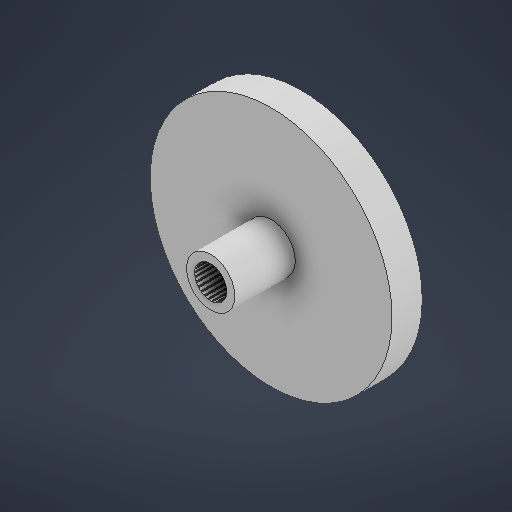
# Autodesk Inventor part: Part7
Saved by Autodesk Inventor 2026.2 (Build 302298000, 298)
## iProperties
Created: 2026-04-16
Part Number: Part7
Material: Generic
Document SubType Name: Modeling
Designer: danda
Density: 1 g/cm^3
Appearance: Default
Author: danda
Autodesk Inventor part; units mm, degrees
ref_plane "YZ Plane" through (0, 0, 0) normal (1, 0, 0) x (0, 1, 0)
ref_plane "XZ Plane" through (0, 0, 0) normal (0, 1, 0) x (-1, 0, 0)
ref_plane "XY Plane" through (0, 0, 0) normal (0, 0, 1) x (1, 0, 0)
sketch "Sketch1" plane through (0, 0, 0) normal (0, 0, 1) x (1, 0, 0)
  line L0 (27.0225, 22.9586) -> (27.3991, 23.1435)
  line L1 (27.3991, 23.1435) -> (27.4189, 23.2234)
  arc A0 (27.4189, 23.2234) -> (27.5041, 23.2788) centre (26.0453, 25.431) ccw
  line L2 (27.5041, 23.2788) -> (27.5858, 23.2643)
  line L3 (27.5858, 23.2643) -> (27.9072, 23.534)
  line L4 (27.9072, 23.534) -> (27.9073, 23.6163)
  arc A1 (27.9073, 23.6163) -> (27.9768, 23.6905) centre (26.0453, 25.431) ccw
  line L5 (27.9768, 23.6905) -> (28.0596, 23.6959)
  line L6 (28.0596, 23.6959) -> (28.3071, 24.0347)
  line L7 (28.3071, 24.0347) -> (28.2875, 24.1147)
  arc A2 (28.2875, 24.1147) -> (28.3372, 24.2033) centre (26.0453, 25.431) ccw
  line L8 (28.3372, 24.2033) -> (28.4163, 24.2284)
  line L9 (28.4163, 24.2284) -> (28.5755, 24.6165)
  line L10 (28.5755, 24.6165) -> (28.5373, 24.6895)
  arc A3 (28.5373, 24.6895) -> (28.5644, 24.7874) centre (26.0453, 25.431) ccw
  line L11 (28.5644, 24.7874) -> (28.6352, 24.8308)
  line L12 (28.6352, 24.8308) -> (28.6969, 25.2457)
  line L13 (28.6969, 25.2457) -> (28.6423, 25.3074)
  arc A4 (28.6423, 25.3074) -> (28.6452, 25.409) centre (26.0453, 25.431) ccw
  line L14 (28.6452, 25.409) -> (28.7035, 25.468)
  line L15 (28.7035, 25.468) -> (28.6642, 25.8857)
  line L16 (28.6642, 25.8857) -> (28.5964, 25.9326)
  arc A5 (28.5964, 25.9326) -> (28.5749, 26.0318) centre (26.0453, 25.431) ccw
  line L17 (28.5749, 26.0318) -> (28.6174, 26.1031)
  line L18 (28.6174, 26.1031) -> (28.4792, 26.4992)
  line L19 (28.4792, 26.4992) -> (28.4023, 26.5285)
  arc A6 (28.4023, 26.5285) -> (28.3576, 26.6197) centre (26.0453, 25.431) ccw
  line L20 (28.3576, 26.6197) -> (28.3818, 26.6991)
  line L21 (28.3818, 26.6991) -> (28.1529, 27.0507)
  line L22 (28.1529, 27.0507) -> (28.0711, 27.0607)
  arc A7 (28.0711, 27.0607) -> (28.0059, 27.1386) centre (26.0453, 25.431) ccw
  line L23 (28.0059, 27.1386) -> (28.0105, 27.2214)
  line L24 (28.0105, 27.2214) -> (27.704, 27.508)
  line L25 (27.704, 27.508) -> (27.6222, 27.4981)
  arc A8 (27.6222, 27.4981) -> (27.5403, 27.5582) centre (26.0453, 25.431) ccw
  line L26 (27.5403, 27.5582) -> (27.5249, 27.6397)
  line L27 (27.5249, 27.6397) -> (27.1587, 27.8446)
  line L28 (27.1587, 27.8446) -> (27.0817, 27.8155)
  arc A9 (27.0817, 27.8155) -> (26.9878, 27.8541) centre (26.0453, 25.431) ccw
  line L29 (26.9878, 27.8541) -> (26.9533, 27.9296)
  line L30 (26.9533, 27.9296) -> (26.5488, 28.0409)
  line L31 (26.5488, 28.0409) -> (26.4809, 27.9942)
  arc A10 (26.4809, 27.9942) -> (26.3805, 28.0093) centre (26.0453, 25.431) ccw
  line L32 (26.3805, 28.0093) -> (26.3289, 28.0743)
  line L33 (26.3289, 28.0743) -> (25.9095, 28.0856)
  line L34 (25.9095, 28.0856) -> (25.8548, 28.024)
  arc A11 (25.8548, 28.024) -> (25.7537, 28.0145) centre (26.0453, 25.431) ccw
  line L35 (25.7537, 28.0145) -> (25.6881, 28.0654)
  line L36 (25.6881, 28.0654) -> (25.2782, 27.9759)
  line L37 (25.2782, 27.9759) -> (25.2398, 27.903)
  arc A12 (25.2398, 27.903) -> (25.1439, 27.8697) centre (26.0453, 25.431) ccw
  line L38 (25.1439, 27.8697) -> (25.068, 27.9033)
  line L39 (25.068, 27.9033) -> (24.6914, 27.7184)
  line L40 (24.6914, 27.7184) -> (24.6716, 27.6385)
  arc A13 (24.6716, 27.6385) -> (24.5864, 27.5831) centre (26.0453, 25.431) ccw
  line L41 (24.5864, 27.5831) -> (24.5047, 27.5976)
  line L42 (24.5047, 27.5976) -> (24.1833, 27.3279)
  line L43 (24.1833, 27.3279) -> (24.1833, 27.2456)
  arc A14 (24.1833, 27.2456) -> (24.1138, 27.1714) centre (26.0453, 25.431) ccw
  line L44 (24.1138, 27.1714) -> (24.031, 27.166)
  line L45 (24.031, 27.166) -> (23.7835, 26.8272)
  line L46 (23.7835, 26.8272) -> (23.8031, 26.7472)
  arc A15 (23.8031, 26.7472) -> (23.7534, 26.6586) centre (26.0453, 25.431) ccw
  line L47 (23.7534, 26.6586) -> (23.6743, 26.6335)
  line L48 (23.6743, 26.6335) -> (23.5151, 26.2454)
  line L49 (23.5151, 26.2454) -> (23.5532, 26.1724)
  arc A16 (23.5532, 26.1724) -> (23.5262, 26.0745) centre (26.0453, 25.431) ccw
  line L50 (23.5262, 26.0745) -> (23.4554, 26.0311)
  line L51 (23.4554, 26.0311) -> (23.3937, 25.6162)
  line L52 (23.3937, 25.6162) -> (23.4482, 25.5545)
  arc A17 (23.4482, 25.5545) -> (23.4454, 25.4529) centre (26.0453, 25.431) ccw
  line L53 (23.4454, 25.4529) -> (23.387, 25.3939)
  line L54 (23.387, 25.3939) -> (23.4264, 24.9762)
  line L55 (23.4264, 24.9762) -> (23.4941, 24.9293)
  arc A18 (23.4941, 24.9293) -> (23.5157, 24.8301) centre (26.0453, 25.431) ccw
  line L56 (23.5157, 24.8301) -> (23.4731, 24.7588)
  line L57 (23.4731, 24.7588) -> (23.6113, 24.3627)
  line L58 (23.6113, 24.3627) -> (23.6883, 24.3334)
  arc A19 (23.6883, 24.3334) -> (23.733, 24.2422) centre (26.0453, 25.431) ccw
  line L59 (23.733, 24.2422) -> (23.7087, 24.1628)
  line L60 (23.7087, 24.1628) -> (23.9377, 23.8112)
  line L61 (23.9377, 23.8112) -> (24.0195, 23.8012)
  arc A20 (24.0195, 23.8012) -> (24.0847, 23.7233) centre (26.0453, 25.431) ccw
  line L62 (24.0847, 23.7233) -> (24.0801, 23.6405)
  line L63 (24.0801, 23.6405) -> (24.3866, 23.3539)
  line L64 (24.3866, 23.3539) -> (24.4683, 23.3638)
  arc A21 (24.4683, 23.3638) -> (24.5503, 23.3037) centre (26.0453, 25.431) ccw
  line L65 (24.5503, 23.3037) -> (24.5657, 23.2222)
  line L66 (24.5657, 23.2222) -> (24.9318, 23.0173)
  line L67 (24.9318, 23.0173) -> (25.0089, 23.0464)
  arc A22 (25.0089, 23.0464) -> (25.1028, 23.0078) centre (26.0453, 25.431) ccw
  line L68 (25.1028, 23.0078) -> (25.1373, 22.9323)
  line L69 (25.1373, 22.9323) -> (25.5418, 22.821)
  line L70 (25.5418, 22.821) -> (25.6096, 22.8677)
  arc A23 (25.6096, 22.8677) -> (25.7101, 22.8526) centre (26.0453, 25.431) ccw
  line L71 (25.7101, 22.8526) -> (25.7616, 22.7876)
  line L72 (25.7616, 22.7876) -> (26.181, 22.7764)
  line L73 (26.181, 22.7764) -> (26.2357, 22.8379)
  arc A24 (26.2357, 22.8379) -> (26.3369, 22.8474) centre (26.0453, 25.431) ccw
  line L74 (26.3369, 22.8474) -> (26.4025, 22.7965)
  line L75 (26.4025, 22.7965) -> (26.8124, 22.886)
  line L76 (26.8124, 22.886) -> (26.8507, 22.9589)
  arc A25 (26.8507, 22.9589) -> (26.9467, 22.9922) centre (26.0453, 25.431) ccw
  line L77 (26.9467, 22.9922) -> (27.0225, 22.9586)
  circle A26 centre (26.0453, 25.431) radius 4
  circle A27 centre (26.0453, 25.431) radius 20
  point P0 (0, 0)
  dimension "d0" = 8
  dimension "d1" = 40
  constraints: 156 end point, 2 centre point, 1 coincident, 79 other
  measures "d0" diameter of A26
  measures "d1" diameter of A27
extrude "Extrusion1" add sketch "Sketch1" along normal blind 10 contours A26
extrude "Extrusion2" add sketch "Sketch1" against normal blind 5 contours A26 | A27
body "Solid1"
